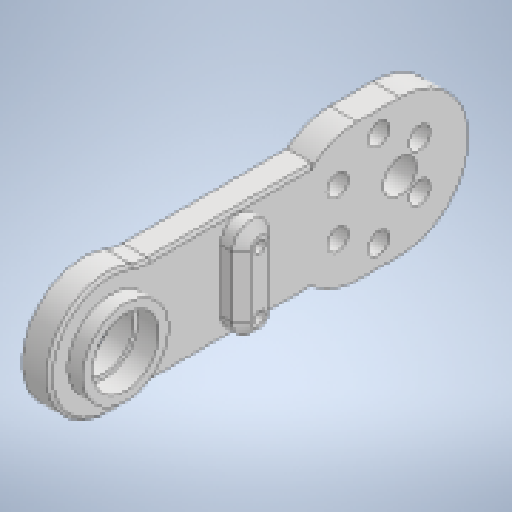
# Autodesk Inventor part: 链轮摇臂
Saved by Autodesk Inventor 2025.1 (Build 291241000, 241)
## iProperties
Created: 2025-08-27
Part Number: 链轮摇臂
Material: 常规
Document SubType Name: Modeling
Designer: Piw
Density: 1 g/cm^3
Appearance: 默认
Author: Piw
Autodesk Inventor part; units mm, degrees
ref_plane "YZ Plane" through (0, 0, 0) normal (1, 0, 0) x (0, 1, 0)
ref_plane "XZ Plane" through (0, 0, 0) normal (0, 1, 0) x (-1, 0, 0)
ref_plane "XY Plane" through (0, 0, 0) normal (0, 0, 1) x (1, 0, 0)
sketch "草图1" plane through (0, 0, 0) normal (1, 0, 0) x (0, 1, 0)
  circle A0 centre (0, 0) radius 9.5
  circle A1 centre (0, 0) radius 20
  dimension "d0" = 19
  dimension "d1" = 40
  constraints: 2 centre point, 2 coincident
  measures "d0" diameter of A0
  measures "d1" diameter of A1
extrude "拉伸1" add sketch "草图1" along normal blind 7
sketch "草图3" plane through (7, 0, 0) normal (1, 0, 0) x (0, 0, -1)
  circle A0 centre (0, 0) radius 11
  circle A1 centre (0, 0) radius 20 projected
  dimension "d4" = 22
  constraints: 1 centre point, 1 coincident
  measures "d4" diameter of A0
extrude "拉伸2" add sketch "草图3" along normal blind 7
sketch "草图4" plane through (0, 0, 0) normal (-1, 0, 0) x (0, 0, 1)
  circle A0 centre (0, 0) radius 20
  line L0 (-9.682458, -17.5) -> (-66.857864, -17.5)
  line L1 (34.622309, 0) -> (-74.086049, 0)
  line L2 (-9.682458, 17.5) -> (-66.857864, 17.5)
  circle A1 centre (-95, 0) radius 5.5
  arc A2 (-72.5, 0) -> (-80.857864, 17.5) centre (-95, 0) ccw construction
  arc A3 (-80.857864, -17.5) -> (-72.5, 0) centre (-95, 0) ccw construction
  line L3 (-95, 0) -> (-81, 0) construction
  line L4 (-95, -22.5) -> (-81, -22.5)
  line L5 (-81, 22.5) -> (-95, 22.5)
  arc A4 (-95, 22.5) -> (-95, -22.5) centre (-95, 0) ccw
  arc A5 (-81, -22.5) -> (-66.857864, -17.5) centre (-81, 0) ccw
  arc A6 (-66.857864, 17.5) -> (-81, 22.5) centre (-81, 0) ccw
  arc A7 (-66.857864, -17.5) -> (-66.857864, 17.5) centre (-81, 0) ccw construction
  circle A8 centre (-88, 0) radius 15.5 construction
  circle A9 centre (-88, 15.5) radius 1.6
  line L6 (-88, 15.5) -> (-88, 0) construction
  circle A10 centre (-101.423394, 7.75) radius 1.6
  circle A11 centre (-101.423394, -7.75) radius 1.6
  circle A12 centre (-88, -15.5) radius 1.6
  circle A13 centre (-74.576606, -7.75) radius 1.6
  circle A14 centre (-74.576606, 7.75) radius 1.6
  point P0 (173.705699, -17.5)
  point P1 (-9.682458, 17.5)
  point P2 (11.5, 0)
  point P3 (-13.5, 0)
  point P4 (-20, 0)
  point P5 (9.682458, -17.5)
  point P6 (20, 0)
  point P7 (9.682458, 17.5)
  dimension "d23" = 31
  dimension "d12" = 95
  dimension "d13" = 35
  dimension "d14" = 11
  dimension "d22" = 45
  dimension "d24" = 3.2
  dimension "d27" = 360
  dimension "d39" = 7
  constraints: 16 end point, 13 centre point, 13 point on circle, 7 tangent, 4 horizontal, 3 point on line, 2 coincident, 2 symmetric about line, 1 midpoint, 1 parallel, 1 perpendicular, 1 vertical alignment, 17 other
  measures "d12" distance of A2.centre point (0, 0)
  measures "d13" distance between parallel lines of L0 L2
  measures "d14" diameter of A1
  measures "d22" diameter of A5
  measures "d24" diameter of A9
  measures "d39" distance of A2.centre point (-88, 0)
extrude "拉伸3" add sketch "草图4" against normal blind 9 contours A0 L0 A5 L4 A4 L5 A6 L2
fillet "圆角1" radius 15 3 edges at (4.5, -17.5, -9.6825) (8, 17.5, -9.6825) (3.5, 17.5, -9.6825)
chamfer "倒角3" distance 2 angle 45 7 edges at (9, 17.5, -39.9241) (9, 21.2132, -73.5) (9, 22.5, -88) (9, 0, -117.5) (9, -22.5, -88) (9, -21.2132, -73.5) (9, -17.5, -39.9241)
sketch "草图5" plane through (9, 0, 0) normal (1, 0, 0) x (0, 0, -1)
  circle A0 centre (88, 15.5) radius 1.6
  circle A1 centre (88, 15.5) radius 3.5
  line L0 (88, 15.5) -> (88, 0) construction
  circle A2 centre (74.576606, 7.75) radius 3.5
  circle A3 centre (74.576606, -7.75) radius 3.5
  circle A4 centre (88, -15.5) radius 3.5
  circle A5 centre (101.423394, -7.75) radius 3.5
  circle A6 centre (101.423394, 7.75) radius 3.5
  point P0 (0, 0)
  dimension "d32" = 7
  dimension "d35" = 360
  constraints: 6 centre point, 2 end point, 1 coincident, 1 vertical, 13 other
  measures "d32" diameter of A1
extrude "拉伸4" cut sketch "草图5" against normal blind 5
sketch "草图6" plane through (14, 0, 0) normal (1, 0, 0) x (0, 0, -1)
  circle A0 centre (0, 0) radius 14
  circle A1 centre (0, 0) radius 20 projected
  dimension "d40" = 28
  constraints: 1 centre point, 1 coincident
  measures "d40" diameter of A0
extrude "拉伸5" cut sketch "草图6" against normal blind 5
sketch "草图7" plane through (0, 0, 0) normal (-1, 0, 0) x (0, 0, 1)
  circle A0 centre (-42, 12) radius 1.9
  line L0 (16.645269, 12) -> (-75.432326, 12)
  line L1 (31.196434, 0) -> (-125.315079, 0) construction
  circle A1 centre (-42, -12) radius 1.9
  point P0 (0, 0)
  dimension "d43" = 3.8
  dimension "d47" = 12
  dimension "d48" = 42
  constraints: 4 end point, 3 horizontal, 2 centre point, 1 point on line, 1 symmetric about line, 1 other
  measures "d43" diameter of A0
  measures "d47" distance from line of L1 A0.centre
  measures "d48" horizontal distance of point (0, 0) A0.centre
extrude "拉伸6" cut sketch "草图7" against normal blind 40
sketch "草图8" plane through (9, 0, 0) normal (1, 0, 0) x (0, 0, -1)
  circle A0 centre (42, 12) radius 1.9 projected
  circle A1 centre (42, -12) radius 1.9 projected
  line L0 (42, 12) -> (42, -12) construction
  line L1 (48, 12) -> (48, -12)
  line L2 (36, -12) -> (36, 12)
  arc A2 (48, 12) -> (36, 12) centre (42, 12) ccw
  arc A3 (36, -12) -> (48, -12) centre (42, -12) ccw
  point P0 (0, 0)
  point P1 (42, 0)
  dimension "d49" = 6
  constraints: 8 end point, 4 point on circle, 4 tangent, 2 centre point, 1 midpoint, 1 parallel, 1 vertical
  measures "d49" radius of A2
extrude "拉伸7" add sketch "草图8" along normal blind 7
chamfer "倒角4" distance 3 angle 45 4 edges at (16, 0, -36) (16, -18, -42) (16, 0, -48) (16, 18, -42)
sketch "草图9" plane through (9, 0, 0) normal (-1, 0, 0) x (0, 0, 1)
  line L0 (-37.126603, 15.5) -> (-46.873397, 15.5)
  line L1 (-37.126603, 15.5) -> (-46.873397, 15.5)
  arc A0 (-37.126603, 15.5) -> (-46.873397, 15.5) centre (-42, 12) ccw
  line L2 (-46.873397, -15.5) -> (-37.126603, -15.5)
  arc A1 (-46.873397, -15.5) -> (-37.126603, -15.5) centre (-42, -12) ccw
  point P0 (0, 0)
extrude "拉伸8" add sketch "草图9" along normal up to surface (9 mm away)
chamfer "倒角5" distance 3 angle 45 5 edges at (9, 0, -36) (9, 13.8384, -47.7114) (9, 13.8384, -36.2886) (9, -13.8384, -36.2886) (9, -13.8384, -47.7114)
equation "\"d45\" = d44"
equation "\"d44\" = 40"
